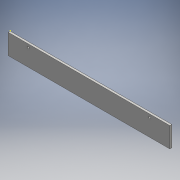
# Autodesk Inventor part: blend_10cm
Saved by Autodesk Inventor 2016 (Build 200138000, 138)
## iProperties
Created: 2016-06-06
Part Number: blend_10cm
Material: Generic
Document SubType Name: Modeling
Designer: Fred
Density: 1 g/cm^3
Appearance: Default
Author: Fred
Autodesk Inventor part; units mm, degrees
ref_plane "YZ Plane" through (0, 0, 0) normal (1, 0, 0) x (0, 1, 0)
ref_plane "XZ Plane" through (0, 0, 0) normal (0, 1, 0) x (-1, 0, 0)
ref_plane "XY Plane" through (0, 0, 0) normal (0, 0, 1) x (1, 0, 0)
sketch "Sketch1" plane through (0, 0, 0) normal (0, 1, 0) x (-1, 0, 0)
  line L0 (0, 0) -> (-800, 0)
  line L1 (-800, 0) -> (-800, -100)
  line L2 (-800, -100) -> (0, -100)
  line L3 (0, -100) -> (0, 0)
  dimension "d0" = 800
  dimension "d1" = 100
  constraints: 8 end point, 2 parallel, 1 horizontal, 1 perpendicular
  measures "d0" distance of L2.end L1.end
  measures "d1" distance of L1.end L0.end
extrude "Extrusion1" add sketch "Sketch1" along normal blind 10
sketch "Sketch2" plane through (0, 10, 0) normal (0, 1, 0) x (1, 0, 0)
  point P0 (0, 0)
sketch "Sketch3" plane through (0, 10, 0) normal (0, 1, 0) x (1, 0, 0)
  circle A0 centre (100, 15) radius 5
  circle A1 centre (700, 15) radius 5
  line L0 (0, 0) -> (800, 0) projected
  line L1 (800, 0) -> (800, 100) projected
  line L2 (0, 100) -> (0, 0) projected
  dimension "d5" = 10
  dimension "d6" = 10
  dimension "d7" = 15
  dimension "d8" = 15
  dimension "d9" = 100
  dimension "d10" = 100
  constraints: 2 centre point
  measures "d5" diameter of A0
  measures "d6" diameter of A1
  measures "d7" distance from line of L0 A0.centre
  measures "d8" distance from line of L0 A1.centre
  measures "d9" distance from line of L1 A1.centre
  measures "d10" distance from line of L2 A0.centre
extrude "Extrusion2" cut sketch "Sketch3" against normal blind 10
equation "\"d6\" = d5"
equation "\"d8\" = d7"
equation "\"d10\" = d9"
body "Solid1"
